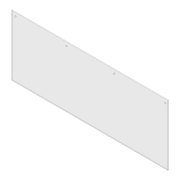
# Autodesk Inventor part: FE-00009
Saved by Autodesk Inventor 2012 (Build 160160000, 160)
## iProperties
Created: 2008-06-02
Part Number: FE-00009
Document SubType Name: Modeling
Designer: mcyr
Density: 1 g/cm^3
Description: Field Plastic "B"
Mass: 3812.28 g
Surface Area: 12234.1 cm^2
Volume: 3812.28 cm^3
Material: Default
Title: FE-00009
Author: mcyr
Autodesk Inventor part; units mm, degrees
ref_plane "YZ Plane" through (0, 0, 0) normal (1, 0, 0) x (0, 1, 0)
ref_plane "XZ Plane" through (0, 0, 0) normal (0, 1, 0) x (-1, 0, 0)
ref_plane "XY Plane" through (0, 0, 0) normal (0, 0, 1) x (1, 0, 0)
sketch "Sketch1" plane through (0, 0, 0) normal (0, 0, 1) x (1, 0, 0)
  line L0 (-47.1537, -0.1898) -> (1197.4463, -0.1898)
  line L1 (1197.4463, -0.1898) -> (1197.4463, 482.4102)
  line L2 (1197.4463, 482.4102) -> (-47.1537, 482.4102)
  line L3 (-47.1537, 482.4102) -> (-47.1537, -0.1898)
  circle A0 centre (-21.7537, 450.6602) radius 4.7625
  circle A1 centre (384.6463, 450.6602) radius 4.7625
  circle A2 centre (765.6463, 450.6602) radius 4.7625
  circle A3 centre (1172.0463, 450.6602) radius 4.7625
  dimension "d0" = 482.6
  dimension "d1" = 1244.6
  dimension "d2" = 9.525
  dimension "d3" = 9.525
  dimension "d4" = 9.525
  dimension "d5" = 9.525
  dimension "d6" = 25.4
  dimension "d7" = 431.8
  dimension "d8" = 812.8
  dimension "d9" = 1219.2
  dimension "d12" = 31.75
  dimension "d13" = 31.75
  dimension "d14" = 31.75
  dimension "d15" = 31.75
  constraints: 8 end point, 4 centre point, 2 parallel, 1 horizontal, 1 perpendicular
  measures "d0" distance of L2.end L0.start
  measures "d1" distance of L0.start L0.end
  measures "d2" diameter of A0
  measures "d3" diameter of A1
  measures "d4" diameter of A2
  measures "d5" diameter of A3
  measures "d6" horizontal distance of L2.end A0.centre
  measures "d7" horizontal distance of A1.centre L2.end
  measures "d8" horizontal distance of A2.centre L2.end
  measures "d9" horizontal distance of A3.centre L2.end
  measures "d12" vertical distance of L2.end A0.centre
  measures "d13" distance from line of L2 A1.centre
  measures "d14" distance from line of L2 A2.centre
  measures "d15" distance from line of L2 A3.centre
extrude "Extrusion1" add sketch "Sketch1" along normal blind 6.35
body "Solid1"
